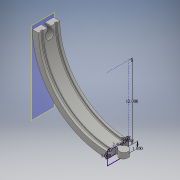
# Autodesk Inventor part: Caufield_Straight_Track
Saved by Autodesk Inventor 2016 (Build 200138000, 138)
## iProperties
Created: 2018-01-11
Part Number: Caufield_Straight_Track
Material: Generic
Document SubType Name: Modeling
Designer: caufield58738
Density: 1 g/cm^3
Appearance: Default
Author: caufield58738
Autodesk Inventor part; units mm, degrees
ref_plane "YZ Plane" through (0, 0, 0) normal (1, 0, 0) x (0, 1, 0)
ref_plane "XZ Plane" through (0, 0, 0) normal (0, 1, 0) x (-1, 0, 0)
ref_plane "XY Plane" through (0, 0, 0) normal (0, 0, 1) x (1, 0, 0)
sketch "Track sketch" plane through (0, 0, 0) normal (0, 0, 1) x (1, 0, 0)
  line L0 (0, 0) -> (86.36, 0)
  line L1 (86.36, 0) -> (86.36, 25.4)
  line L2 (0, 25.4) -> (0, 0)
  line L3 (19.05, 25.4) -> (19.05, 20.6375)
  line L4 (19.05, 20.6375) -> (10.16, 20.6375)
  line L5 (10.16, 20.6375) -> (10.16, 25.4)
  line L6 (43.18, 25.4) -> (43.18, 0) construction
  line L7 (67.31, 25.4) -> (67.31, 20.6375)
  line L8 (67.31, 20.6375) -> (76.2, 20.6375)
  line L9 (76.2, 20.6375) -> (76.2, 25.4)
  line L10 (10.16, 25.4) -> (0, 25.4)
  line L11 (86.36, 25.4) -> (76.2, 25.4)
  line L12 (67.31, 25.4) -> (19.05, 25.4)
  line L13 (0, 0) -> (0, 304.8) construction
  line L14 (0, 304.8) -> (86.36, 304.8) construction
  line L15 (0, 0) -> (0, -25.4)
  line L16 (0, -25.4) -> (86.36, -25.4)
  line L17 (86.36, -25.4) -> (86.36, 0)
  dimension "d0" = 86.36
  dimension "d1" = 25.4
  dimension "d2" = 19.05
  dimension "d3" = 10.16
  dimension "d6" = 4.7625
  dimension "d23" = 304.8
  dimension "d47" = 25.4
  constraints: 36 end point, 5 parallel, 4 symmetric about line, 3 perpendicular, 2 collinear, 2 horizontal, 2 midpoint, 2 vertical
  measures "d0" distance of L2.start L1.end
  measures "d1" distance of L1.end L0.end
  measures "d2" distance between parallel lines of L3 L2
  measures "d3" distance between parallel lines of L5 L2
  measures "d6" distance of L4.end L5.end
  measures "d23" distance of L0.start L13.end
  measures "d47" distance between parallel lines of L16 L0
revolve "Revolution1" add sketch "Track sketch" angle 90 about axis through (0, 304.8, 0) along (-1, 0, 0) contours L2 L10 L5 L4 L3 L12 L7 L8 L9 L11 L1 L0
sketch "Sketch3" plane through (0, 0, 0) normal (0, 1, 0) x (-1, 0, 0)
  line L0 (-19.50225, 0) -> (-66.85775, 0)
  line L1 (-43.18, 304.8) -> (-43.18, 0) construction
  line L2 (-43.18, 0) -> (-43.18, -37.562444) construction
  arc A0 (-52.968989, -10.557355) -> (-33.391011, -10.557355) centre (-43.18, -25.4) ccw
  line L3 (-50.8, 0) -> (-35.56, 0)
  line L4 (-35.56, 0) -> (-35.56, -6.528638)
  line L5 (-35.56, -9.335629) -> (-50.8, -9.335629) construction
  line L6 (-50.8, -6.528638) -> (-50.8, 0)
  arc A1 (-52.968989, -10.557355) -> (-50.8, -6.528638) centre (-55.626, -6.528638) ccw
  arc A2 (-35.56, -6.528638) -> (-33.391011, -10.557355) centre (-30.734, -6.528638) ccw
  line L7 (0, 0) -> (-86.36, 0)
  line L8 (-86.36, 0) -> (-86.36, 304.8)
  line L9 (0, 304.8) -> (-86.36, 304.8)
  line L10 (0, 0) -> (0, 304.8)
  line L11 (0, 0) -> (-86.36, 0)
  line L12 (0, 304.8) -> (-86.36, 304.8) construction
  line L13 (-43.18, 304.8) -> (-43.18, 65.498651) construction
  point P0 (-43.18, 279.4)
  dimension "d25" = 279.4
  dimension "d26" = 35.56
  dimension "d27" = 25.4
  dimension "d28" = 15.24
  dimension "d29" = 4.826
  dimension "d32" = 86.36
  dimension "d33" = 43.18
  dimension "d34" = 43.18
  dimension "d35" = 25.4
  constraints: 16 end point, 8 point on circle, 6 point on line, 4 tangent, 3 centre point, 2 midpoint, 2 parallel, 1 collinear, 1 equal radius, 1 horizontal, 1 perpendicular, 1 vertical
  measures "d25" distance from line of L0 point (-43.18, 279.4)
  measures "d26" diameter of A0
  measures "d27" distance from line of L0 A0.centre
  measures "d28" distance of L5.end L5.start
  measures "d29" radius of A1
  measures "d32" distance of L7.end L11.start
  measures "d33" distance from line of L8 L13.end
  measures "d34" distance from line of L11.start L2
  measures "d35" vertical distance of L11.start A0.centre
extrude "Extrusion4" add sketch "Sketch3" along normal blind 25.4 contours L4 A2 A0 A1 L6 L0
ref_plane "Work Plane1" through (0, 304.8, 304.8) normal (0, 0, 1) x (1, 0, 0)
sketch "Sketch4" plane through (0, 304.8, 304.8) normal (0, 0, 1) x (1, 0, 0)
  line L0 (0, -304.8) -> (35.56, -304.8)
  line L1 (35.56, -304.8) -> (50.8, -304.8)
  line L2 (50.8, -304.8) -> (86.36, -304.8)
  line L3 (86.36, -304.8) -> (86.36, 0)
  line L4 (0, 0) -> (86.36, 0)
  line L5 (0, -304.8) -> (0, 0)
  line L6 (67.31, 0) -> (19.05, 0)
  line L7 (43.18, 304.8) -> (43.18, 0) construction
  line L8 (43.18, 0) -> (43.18, -37.562444) construction
  arc A0 (33.391011, -10.557355) -> (52.968989, -10.557355) centre (43.18, -25.4) ccw
  line L9 (35.56, 0) -> (50.8, 0)
  line L10 (50.8, 0) -> (50.8, -6.528638)
  line L11 (50.8, -9.335629) -> (35.56, -9.335629) construction
  line L12 (35.56, -6.528638) -> (35.56, 0)
  arc A1 (33.391011, -10.557355) -> (35.56, -6.528638) centre (30.734, -6.528638) ccw
  arc A2 (50.8, -6.528638) -> (52.968989, -10.557355) centre (55.626, -6.528638) ccw
  point P0 (43.18, 279.4)
  dimension "d38" = 279.4
  dimension "d39" = 35.56
  dimension "d40" = 25.4
  dimension "d41" = 15.24
  dimension "d42" = 4.826
  dimension "d43" = 43.18
  dimension "d44" = 25.4
  constraints: 14 end point, 8 point on circle, 5 point on line, 4 tangent, 3 centre point, 2 parallel, 1 equal radius, 1 horizontal, 1 midpoint, 1 perpendicular, 1 vertical
  measures "d38" distance from line of L6 point (43.18, 279.4)
  measures "d39" diameter of A0
  measures "d40" distance from line of L6 A0.centre
  measures "d41" distance of L11.end L11.start
  measures "d42" radius of A1
  measures "d43" distance between parallel lines of L5 L8
  measures "d44" vertical distance of L4.start A0.centre
extrude "Extrusion5" cut sketch "Sketch4" against normal blind 50.8 contours L4 L10 A2 A0 A1 L12
sketch "Track sketch outline for Revolution2" plane through (0, 0, 0) normal (0, 0, 1) x (1, 0, 0)
  line L0 (86.36, 0) -> (0, 0)
  line L1 (86.36, -25.4) -> (86.36, 0)
  line L2 (0, -25.4) -> (86.36, -25.4)
  line L3 (0, 0) -> (0, -25.4)
revolve "Revolution2" cut sketch "Track sketch outline for Revolution2" angle 360 about axis through (0, 304.8, 0) along (1, 0, 0)
body "Solid2"
